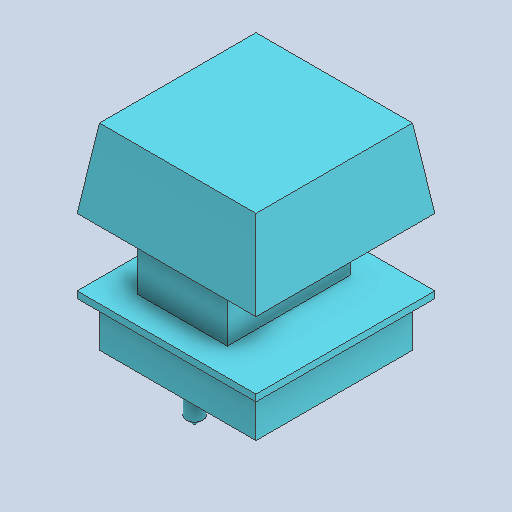
# Autodesk Inventor part: switch
Saved by Autodesk Inventor 2025.2 (Build 292293000, 293)
## iProperties
Created: 2024-03-12
Part Number: switch
Material: Generic
Document SubType Name: Modeling
Designer: mirun
Density: 1 g/cm^3
Appearance: Default
Author: mirun
Autodesk Inventor part; units mm, degrees
ref_plane "YZ Plane" through (0, 0, 0) normal (1, 0, 0) x (0, 1, 0)
ref_plane "XZ Plane" through (0, 0, 0) normal (0, 1, 0) x (-1, 0, 0)
ref_plane "XY Plane" through (0, 0, 0) normal (0, 0, 1) x (1, 0, 0)
sketch "Sketch1" plane through (0, 0, 0) normal (0, 1, 0) x (-1, 0, 0)
  line L0 (-7, 7) -> (7, 7)
  line L1 (7, 7) -> (7, -7)
  line L2 (7, -7) -> (-7, -7)
  line L3 (-7, -7) -> (-7, 7)
  line L4 (-7, 7) -> (7, -7) construction
  line L5 (7, 7) -> (-7, -7) construction
  point P0 (0, 0)
  dimension "d0" = 14
  dimension "d1" = 14
  constraints: 12 end point, 2 midpoint, 2 parallel, 1 horizontal, 1 perpendicular
  measures "d0" distance of L1.end L2.end
  measures "d1" distance of L0.end L1.end
extrude "Extrusion1" add sketch "Sketch1" along normal blind 4
sketch "Sketch2" plane through (0, 4, 0) normal (0, 1, 0) x (1, 0, 0)
  line L0 (8, 8) -> (-8, 8)
  line L1 (-8, 8) -> (-8, -8)
  line L2 (-8, -8) -> (8, -8)
  line L3 (8, -8) -> (8, 8)
  line L4 (8, 8) -> (-8, -8) construction
  line L5 (-8, 8) -> (8, -8) construction
  point P0 (0, 0)
  dimension "d4" = 16
  dimension "d5" = 16
  constraints: 12 end point, 2 midpoint, 2 parallel, 1 horizontal, 1 perpendicular
  measures "d4" distance of L2.end L1.end
  measures "d5" distance of L1.end L0.end
extrude "Extrusion2" add sketch "Sketch2" along normal blind 0.6
sketch "Sketch3" plane through (0, 4.6, 0) normal (0, 1, 0) x (1, 0, 0)
  line L0 (3, -5.5611) -> (-5, -5.5611)
  line L1 (-5, -5.5611) -> (-5, 5.4389)
  line L2 (-5, 5.4389) -> (3, 5.4389)
  line L3 (3, 5.4389) -> (3, -5.5611)
  line L4 (3, -5.5611) -> (-5, 5.4389) construction
  line L5 (-5, -5.5611) -> (3, 5.4389) construction
  point P0 (0, 0)
  point P1 (-1, -0.0611)
  dimension "d8" = 8
  dimension "d9" = 11
  constraints: 12 end point, 2 midpoint, 2 parallel, 1 horizontal, 1 perpendicular
  measures "d8" distance of L1.end L2.end
  measures "d9" distance of L0.end L1.end
extrude "Extrusion3" add sketch "Sketch3" along normal blind 6
sketch "Sketch4" plane through (0, 10.6, 0) normal (0, 1, 0) x (1, 0, 0)
  line L0 (8, -8) -> (-8, -8)
  line L1 (-8, -8) -> (-8, 8)
  line L2 (-8, 8) -> (8, 8)
  line L3 (8, 8) -> (8, -8)
  line L4 (8, -8) -> (-8, 8) construction
  line L5 (-8, -8) -> (8, 8) construction
  point P0 (0, 0)
  dimension "d12" = 16
  dimension "d13" = 16
  constraints: 12 end point, 2 midpoint, 2 parallel, 1 horizontal, 1 perpendicular
  measures "d12" distance of L1.end L2.end
  measures "d13" distance of L0.end L1.end
extrude "Extrusion4" add sketch "Sketch4" along normal blind 7
chamfer "Chamfer1" distance 1 distance2 7 4 edges at (8, 17.6, 0) (0, 17.6, 8) (0, 17.6, -8) (-8, 17.6, 0) measured on face at (-2.6667, 17.6, 2.6667)
sketch "Sketch5" plane through (0, 0, 0) normal (0, -1, 0) x (1, 0, 0)
  circle A0 centre (0, 0) radius 2
  line L0 (-5, -5.4389) -> (3, -5.4389) construction
  line L1 (0, 0) -> (0, -11)
  line L2 (0, 0) -> (4.5527, 0)
  circle A1 centre (0, -5.5) radius 0.75
  circle A2 centre (0, 5.5) radius 0.75
  dimension "d19" = 4
  dimension "d22" = 1.5
  dimension "d23" = 5.5
  constraints: 4 end point, 3 centre point, 1 coincident, 1 horizontal, 1 midpoint, 1 symmetric about line, 1 vertical, 1 other
  measures "d19" diameter of A0
  measures "d22" diameter of A1
  measures "d23" distance of point (0, 0) A1.centre
extrude "Extrusion5" add sketch "Sketch5" along normal blind 3
chamfer "Chamfer2" distance 0.7 angle 45 3 edges at (-2, -3, 0) (-0.75, -3, 5.5) (-0.75, -3, -5.5)
body "Solid1"
